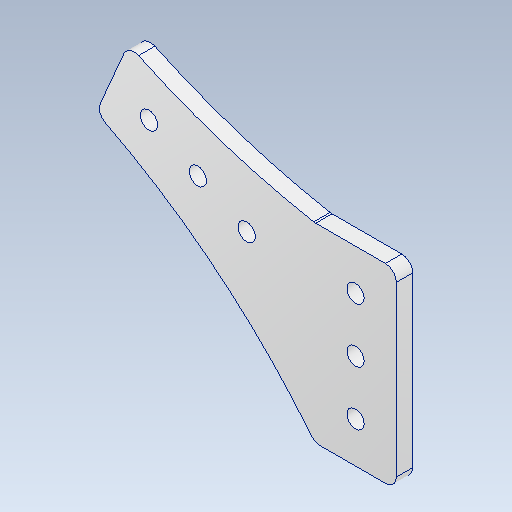
# Autodesk Inventor part: オムニ_固定具寸法不明
Saved by Autodesk Inventor 2021 (Build 250183000, 183)
## iProperties
Created: 2022-02-03
Part Number: オムニ_固定具寸法不明
Material: アルミニウム 6061
Document SubType Name: Modeling
Designer: hirohumi
Density: 2.7 g/cm^3
Appearance: アルミニウム - フラット
Mass: 10.6557 g
Surface Area: 33.0622 cm^2
Volume: 3.94655 cm^3
Author: hirohumi
Autodesk Inventor part; units mm, degrees
ref_plane "YZ Plane" through (0, 0, 0) normal (1, 0, 0) x (0, 1, 0)
ref_plane "XZ Plane" through (0, 0, 0) normal (0, 1, 0) x (-1, 0, 0)
ref_plane "XY Plane" through (0, 0, 0) normal (0, 0, 1) x (1, 0, 0)
sketch "スケッチ1" plane through (0, 0, 0) normal (0, 0, 1) x (1, 0, 0)
  circle A0 centre (7.5, 45) radius 1.6 projected
  circle A1 centre (7.5, 55) radius 1.6 projected
  circle A2 centre (7.5, 65) radius 1.6 projected
  circle A3 centre (-313, 207) radius 1.6 projected
  circle A4 centre (-303, 207) radius 1.6 projected
  circle A5 centre (-293, 207) radius 1.6 projected
  line L0 (7.5, 55) -> (-303, 207) construction
  line L1 (-269.6677, 199.0332) -> (-0.2209, 67.1301) construction
  line L2 (-0.2209, 67.1301) -> (-6.816, 53.6577) construction
  line L3 (-6.816, 53.6577) -> (-276.2628, 185.5608) construction
  line L4 (-276.2628, 185.5608) -> (-269.6677, 199.0332)
  line L5 (-269.6677, 199.0332) -> (-6.816, 53.6577) construction
  line L6 (-0.2209, 67.1301) -> (-276.2628, 185.5608) construction
  circle A6 centre (-12.5, 64.7907) radius 1.6
  circle A7 centre (-21.4816, 69.1874) radius 1.6
  circle A8 centre (-30.4631, 73.5842) radius 1.6
  line L7 (0, 37.5) -> (15, 37.5)
  line L8 (15, 37.5) -> (15, 72.5)
  line L9 (15, 72.5) -> (0, 72.5)
  arc A9 (0, 37.5) -> (-40.1685, 69.9848) centre (-91.1179, -34.0928) ccw
  line L10 (-40.1685, 69.9848) -> (-34.2469, 83.7869)
  arc A10 (-34.2469, 83.7869) -> (0, 72.5) centre (23.8497, 202.4647) ccw
  point P0 (0, 0)
  point P1 (-138.2418, 126.3454)
  dimension "d0" = 300
  dimension "d1" = 15
  dimension "d2" = 3.2
  dimension "d3" = 3.2
  dimension "d4" = 3.2
  dimension "d5" = 10
  dimension "d6" = 10
  dimension "d7" = 10
  dimension "d8" = 20
  dimension "d9" = 7.5
  dimension "d10" = 7.5
  dimension "d11" = 7.5
  dimension "d13" = 7.5
  dimension "d14" = 7.5
  dimension "d15" = 15
  constraints: 22 end point, 6 point on line, 5 centre point, 4 point on circle, 3 parallel, 3 perpendicular, 2 midpoint, 2 tangent, 1 horizontal, 1 vertical
  measures "d0" distance of L2.end L3.end
  measures "d1" distance of L1.end L2.end
  measures "d2" diameter of A6
  measures "d3" diameter of A7
  measures "d4" diameter of A8
  measures "d5" distance of A7.centre A8.centre
  measures "d6" distance of A6.centre A7.centre
  measures "d7" distance from line of L2 A6.centre
  measures "d8" horizontal distance of A2.centre A6.centre
  measures "d9" distance from line of A2.centre L9
  measures "d10" distance from line of L8 A2.centre
  measures "d11" distance from line of A0.centre L7
  measures "d13" horizontal distance of A2.centre L9.end
  measures "d14" distance from line of A8.centre L10
  measures "d15" distance of L7.start L7.end
extrude "押し出し1" add sketch "スケッチ1" along normal blind 3 contours A9 L10 A10 L9 L8 L7
fillet "フィレット1" radius 2 6 edges at (0, 37.5, 1.5) (15, 37.5, 1.5) (15, 72.5, 1.5) (0, 72.5, 1.5) (-40.1685, 69.9848, 1.5) (-34.2469, 83.7869, 1.5)
